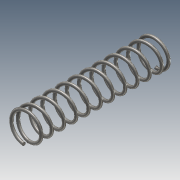
# Autodesk Inventor part: Mola do Captador
Saved by Autodesk Inventor 2016 (Build 200138000, 138)
## iProperties
Created: 2018-12-10
Part Number: Mola do Captador
Material: Generic
Document SubType Name: Modeling
Designer: lesly
Density: 1 g/cm^3
Appearance: Steel - Polished
Author: lesly
Autodesk Inventor part; units mm, degrees
ref_plane "YZ Plane" through (0, 0, 0) normal (1, 0, 0) x (0, 1, 0)
ref_plane "XZ Plane" through (0, 0, 0) normal (0, 1, 0) x (-1, 0, 0)
ref_plane "XY Plane" through (0, 0, 0) normal (0, 0, 1) x (1, 0, 0)
sketch "Sketch2" plane through (0, 0, 0) normal (1, 0, 0) x (0, 1, 0)
  line L0 (0, 0) -> (0, -2.25) construction
  circle A0 centre (0, -2.25) radius 0.25
  dimension "d0" = 2.25
  dimension "d1" = 0.5
  constraints: 2 end point, 1 centre point, 1 coincident, 1 vertical
  measures "d0" distance of L0.start L0.end
  measures "d1" diameter of A0
coil "Coil1" sketch "Sketch2" operation add axis through (0, -10, 0) along (0, 1, 0) pitch 2 turns 10 hand right
sketch "Sketch3" plane through (0, 20, -2.25) normal (-1, 0, 0) x (0, 0, 1)
  circle A0 centre (0, 0) radius 0.25 projected
  point P0 (2.25, -20)
  point P1 (0, 0.25)
  constraints: 1 vertical alignment
coil "Coil2" sketch "Sketch3" operation add axis through (0, -10, 0) along (0, 1, 0) pitch 0.8 turns 1 hand right
sketch "Sketch4" plane through (0, 0, -2.25) normal (1, 0, 0) x (0, 0, -1)
  circle A0 centre (0, 0) radius 0.25 projected
  point P0 (-2.25, 0)
  point P1 (0, 0.25)
  constraints: 1 vertical alignment
coil "Coil3" sketch "Sketch4" operation add axis through (0, -10, 0) along (0, -1, 0) pitch 0.8 turns 1 hand right
body "Solid1"
